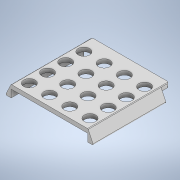
# Autodesk Inventor part: flange2_grip_support
Saved by Autodesk Inventor 2020 (Build 240168000, 168)
## iProperties
Created: 2019-10-19
Part Number: flange2_grip_support
Material: Generic
Document SubType Name: Modeling
Designer: ayad493
Density: 1 g/cm^3
Appearance: Default
Author: ayad493
Autodesk Inventor part; units mm, degrees
ref_plane "YZ Plane" through (0, 0, 0) normal (1, 0, 0) x (0, 1, 0)
ref_plane "XZ Plane" through (0, 0, 0) normal (0, 1, 0) x (-1, 0, 0)
ref_plane "XY Plane" through (0, 0, 0) normal (0, 0, 1) x (1, 0, 0)
sketch "Sketch1" plane through (0, 0, 0) normal (0, 0, 1) x (1, 0, 0)
  line L0 (0, 0) -> (19, 0)
  line L1 (19, 0) -> (20.4, 0)
  line L2 (0, 0) -> (-1.4, 0)
  line L3 (0, 0) -> (0, 1.9)
  line L4 (-1.4, 0) -> (0, 2.9)
  line L5 (19, 0) -> (19, 1.9)
  line L6 (19, 2.9) -> (20.4, 0)
  line L7 (0, 2.9) -> (19, 2.9)
  line L8 (0, 1.9) -> (19, 1.9)
  dimension "d0" = 19
  dimension "d1" = 1.4
  dimension "d2" = 1.4
  dimension "d3" = 2.9
  dimension "d4" = 2.9
  dimension "d5" = 1
  constraints: 18 end point, 2 horizontal, 2 vertical, 1 parallel, 1 point on line
  measures "d0" distance of L0.start L0.end
  measures "d1" distance of L0.end L1.end
  measures "d2" distance of L0.start L2.end
  measures "d3" distance of L0.start L4.end
  measures "d4" distance of L0.end L6.start
  measures "d5" distance between parallel lines of L7 L8
extrude "Extrusion1" add sketch "Sketch1" along normal blind 20 contours L2 L4 L7 L6 L1 L5 L8 L3
fillet "Fillet1" radius 0.2 4 edges at (0, 2.9, 10) (19, 2.9, 10) (20.4, 0, 10) (-1.4, 0, 10)
sketch "Sketch2" plane through (0, 1.9, 0) normal (0, -1, 0) x (1, 0, 0)
  line L0 (-1.2814, 0) -> (-1.2814, 20) projected
  line L1 (0, 0) -> (0, 20) projected
  line L2 (-1.2814, 0) -> (0, 0)
  line L3 (0, 0) -> (0, 2)
  line L4 (0, 2) -> (-1.2814, 2)
  line L5 (-1.2814, 2) -> (-1.2814, 0)
  line L6 (19, 0) -> (19, 20) projected
  line L7 (20.2814, 0) -> (20.2814, 20) projected
  line L8 (19, 0) -> (20.2814, 0)
  line L9 (20.2814, 0) -> (20.2814, 2)
  line L10 (20.2814, 2) -> (19, 2)
  line L11 (19, 2) -> (19, 0)
  dimension "d9" = 2
  dimension "d10" = 2
  constraints: 16 end point, 4 parallel, 3 point on line, 2 horizontal, 2 perpendicular
  measures "d9" distance of L3.end L2.end
  measures "d10" distance of L9.end L8.end
extrude "Extrusion2" cut sketch "Sketch2" along normal blind 20
sketch "Sketch3" plane through (0.1255, 2.9, 0) normal (0, 1, 0) x (1, 0, 0)
  line L0 (-0.1255, -2) -> (-0.6083, -2) projected
  line L1 (18.7489, 0) -> (18.7489, -20) projected
  line L2 (-0.1255, -2) -> (18.7489, -2)
  line L3 (18.7489, -2) -> (18.7489, -20)
  line L4 (18.7489, -20) -> (-0.1255, -20)
  line L5 (-0.1255, -20) -> (-0.1255, -2)
  line L6 (-0.1255, -2) -> (-0.1255, -20) projected
  line L7 (-0.1255, -2) -> (1.8745, -2)
  line L8 (1.8745, -2) -> (1.8745, -4)
  line L9 (0.8745, -5) -> (2.8745, -5)
  line L10 (2.8745, -5) -> (2.8745, -3)
  line L11 (2.8745, -3) -> (0.8745, -3)
  line L12 (0.8745, -3) -> (0.8745, -5)
  line L13 (0.8745, -5) -> (2.8745, -3) construction
  line L14 (2.8745, -5) -> (0.8745, -3) construction
  line L15 (7.8745, -3) -> (5.8745, -3)
  line L16 (5.8745, -3) -> (5.8745, -5)
  line L17 (7.8745, -5) -> (7.8745, -3)
  line L18 (5.8745, -5) -> (7.8745, -5)
  line L19 (12.8745, -3) -> (10.8745, -3)
  line L20 (10.8745, -3) -> (10.8745, -5)
  line L21 (12.8745, -5) -> (12.8745, -3)
  line L22 (10.8745, -5) -> (12.8745, -5)
  line L23 (17.8745, -3) -> (15.8745, -3)
  line L24 (15.8745, -3) -> (15.8745, -5)
  line L25 (17.8745, -5) -> (17.8745, -3)
  line L26 (15.8745, -5) -> (17.8745, -5)
  line L27 (2.8745, -7.5) -> (0.8745, -7.5)
  line L28 (0.8745, -7.5) -> (0.8745, -9.5)
  line L29 (2.8745, -9.5) -> (2.8745, -7.5)
  line L30 (0.8745, -9.5) -> (2.8745, -9.5)
  line L31 (7.8745, -7.5) -> (5.8745, -7.5)
  line L32 (5.8745, -7.5) -> (5.8745, -9.5)
  line L33 (7.8745, -9.5) -> (7.8745, -7.5)
  line L34 (5.8745, -9.5) -> (7.8745, -9.5)
  line L35 (12.8745, -7.5) -> (10.8745, -7.5)
  line L36 (10.8745, -7.5) -> (10.8745, -9.5)
  line L37 (12.8745, -9.5) -> (12.8745, -7.5)
  line L38 (10.8745, -9.5) -> (12.8745, -9.5)
  line L39 (17.8745, -7.5) -> (15.8745, -7.5)
  line L40 (15.8745, -7.5) -> (15.8745, -9.5)
  line L41 (17.8745, -9.5) -> (17.8745, -7.5)
  line L42 (15.8745, -9.5) -> (17.8745, -9.5)
  line L43 (2.8745, -12) -> (0.8745, -12)
  line L44 (0.8745, -12) -> (0.8745, -14)
  line L45 (2.8745, -14) -> (2.8745, -12)
  line L46 (0.8745, -14) -> (2.8745, -14)
  line L47 (7.8745, -12) -> (5.8745, -12)
  line L48 (5.8745, -12) -> (5.8745, -14)
  line L49 (7.8745, -14) -> (7.8745, -12)
  line L50 (5.8745, -14) -> (7.8745, -14)
  line L51 (12.8745, -12) -> (10.8745, -12)
  line L52 (10.8745, -12) -> (10.8745, -14)
  line L53 (12.8745, -14) -> (12.8745, -12)
  line L54 (10.8745, -14) -> (12.8745, -14)
  line L55 (17.8745, -12) -> (15.8745, -12)
  line L56 (15.8745, -12) -> (15.8745, -14)
  line L57 (17.8745, -14) -> (17.8745, -12)
  line L58 (15.8745, -14) -> (17.8745, -14)
  line L59 (2.8745, -16.5) -> (0.8745, -16.5)
  line L60 (0.8745, -16.5) -> (0.8745, -18.5)
  line L61 (2.8745, -18.5) -> (2.8745, -16.5)
  line L62 (0.8745, -18.5) -> (2.8745, -18.5)
  line L63 (7.8745, -16.5) -> (5.8745, -16.5)
  line L64 (5.8745, -16.5) -> (5.8745, -18.5)
  line L65 (7.8745, -18.5) -> (7.8745, -16.5)
  line L66 (5.8745, -18.5) -> (7.8745, -18.5)
  line L67 (12.8745, -16.5) -> (10.8745, -16.5)
  line L68 (10.8745, -16.5) -> (10.8745, -18.5)
  line L69 (12.8745, -18.5) -> (12.8745, -16.5)
  line L70 (10.8745, -18.5) -> (12.8745, -18.5)
  line L71 (17.8745, -16.5) -> (15.8745, -16.5)
  line L72 (15.8745, -16.5) -> (15.8745, -18.5)
  line L73 (17.8745, -18.5) -> (17.8745, -16.5)
  line L74 (15.8745, -18.5) -> (17.8745, -18.5)
  circle A0 centre (1.8745, -4) radius 1.4142
  circle A1 centre (6.8745, -4) radius 1.4142
  circle A2 centre (11.8745, -4) radius 1.4142
  circle A3 centre (16.8745, -4) radius 1.4142
  circle A4 centre (1.8745, -8.5) radius 1.4142
  circle A5 centre (6.8745, -8.5) radius 1.4142
  circle A6 centre (11.8745, -8.5) radius 1.4142
  circle A7 centre (16.8745, -8.5) radius 1.4142
  circle A8 centre (1.8745, -13) radius 1.4142
  circle A9 centre (6.8745, -13) radius 1.4142
  circle A10 centre (11.8745, -13) radius 1.4142
  circle A11 centre (16.8745, -13) radius 1.4142
  circle A12 centre (1.8745, -17.5) radius 1.4142
  circle A13 centre (6.8745, -17.5) radius 1.4142
  circle A14 centre (11.8745, -17.5) radius 1.4142
  circle A15 centre (16.8745, -17.5) radius 1.4142
  point P0 (-0.1255, 0)
  dimension "d13" = 2
  dimension "d14" = 2
  dimension "d15" = 2
  dimension "d16" = 2
  dimension "d19" = 5
  dimension "d22" = 4.5
  dimension "d32" = 5
  dimension "d35" = 4.5
  constraints: 144 end point, 16 centre point, 4 horizontal, 4 parallel, 3 perpendicular, 2 midpoint, 2 vertical, 1 coincident, 1 point on line, 150 other
  measures "d13" distance of L0.start L7.end
  measures "d14" distance of L7.end L8.end
  measures "d15" distance of L11.end L10.end
  measures "d16" distance of L10.end L9.end
  measures "d19" distance of L10.end L15.start
  measures "d22" distance of L10.end L27.start
  measures "d32" distance of A0.centre A1.centre
  measures "d35" distance of A0.centre A4.centre
extrude "Extrusion3" cut sketch "Sketch3" against normal through all contours A0 L11 L8 | L8 L11 A0 | L11 L10 L9 L12 | A0 L10 | L12 A0 | A0 L9 | L17 L18 L16 L15 | A1 L17 | L15 A1 | L16 A1 | A1 L18 | L21 L22 L20 L19 | A2 L21 | L19 A2 | L20 A2 | A2 L22 | L25 L26 L24 L23 | A3 L25 | L23 A3 | L24 A3 | A3 L26 | L29 L30 L28 L27 | A4 L29 | L27 A4 | L28 A4 | A4 L30 | L33 L34 L32 L31 | A5 L33 | L31 A5 | L32 A5 | A5 L34 | L37 L38 L36 L35 | A6 L37 | L35 A6 | L36 A6 | A6 L38 | L41 L42 L40 L39 | A7 L41 | L39 A7 | L40 A7 | A7 L42 | L45 L46 L44 L43 | A8 L45 | L43 A8 | L44 A8 | A8 L46 | L49 L50 L48 L47 | A9 L49 | L47 A9 | L48 A9 | A9 L50 | L53 L54 L52 L51 | A10 L53 | L51 A10 | L52 A10 | A10 L54 | L57 L58 L56 L55 | A11 L57 | L55 A11 | L56 A11 | A11 L58 | L61 L62 L60 L59 | A12 L61 | L59 A12 | L60 A12 | A12 L62 | L65 L66 L64 L63 | A13 L65 | L63 A13 | L64 A13 | A13 L66 | L69 L70 L68 L67 | A14 L69 | L67 A14 | L68 A14 | A14 L70 | L73 L74 L72 L71 | A15 L73 | L71 A15 | L72 A15 | A15 L74
sketch "Sketch4" plane through (-0.4828, 1.9, 0) normal (0, -1, 0) x (1, 0, 0)
  line L0 (0, 0) -> (0, 2) projected
  line L1 (0, 2) -> (0.4828, 2)
  line L2 (0.4828, 2) -> (0.4828, 0)
  line L3 (0.4828, 0) -> (0, 0)
  line L4 (0, 0) -> (0, 2)
  line L5 (19.9655, 2) -> (19.9655, 0) projected
  line L6 (19.9655, 0) -> (19.5373, 0) projected
  line L7 (19.9655, 2) -> (19.5373, 2)
  line L8 (19.5373, 2) -> (19.5373, 0)
  line L9 (19.5373, 0) -> (19.9655, 0)
  line L10 (19.9655, 0) -> (19.9655, 2)
  constraints: 16 end point, 4 parallel, 2 horizontal, 2 perpendicular
extrude "Extrusion4" cut sketch "Sketch4" against normal blind 20
fillet "Fillet2" radius 0.5 2 edges at (19.0546, 2.3435, 0) (0, 2.3778, 0)
body "Solid1"
